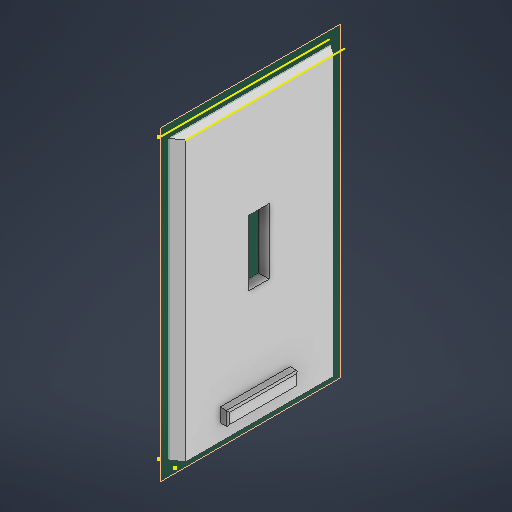
# Autodesk Inventor part: Part2
Saved by Autodesk Inventor 2026.1 (Build 301233000, 233)
## iProperties
Created: 2025-08-25
Part Number: Part2
Material: Generic
Document SubType Name: Modeling
Designer: usman
Density: 1 g/cm^3
Appearance: Default
Author: usman
Autodesk Inventor part; units mm, degrees
ref_plane "YZ Plane" through (0, 0, 0) normal (1, 0, 0) x (0, 1, 0)
ref_plane "XZ Plane" through (0, 0, 0) normal (0, 1, 0) x (-1, 0, 0)
ref_plane "XY Plane" through (0, 0, 0) normal (0, 0, 1) x (1, 0, 0)
sketch "Sketch1" plane through (0, 0, 0) normal (1, 0, 0) x (0, 1, 0)
  line L0 (0, 0) -> (178.9, 0)
  line L1 (178.9, 0) -> (178.9, -109)
  line L2 (178.9, -109) -> (0, -109)
  line L3 (0, -109) -> (0, 0)
  dimension "d0" = 178.9
  dimension "d1" = 109
  constraints: 8 end point, 2 parallel, 1 horizontal, 1 perpendicular
  measures "d0" distance of L1.end L2.end
  measures "d1" distance of L0.end L1.end
extrude "Extrusion1" add sketch "Sketch1" along normal blind 10
sketch "Sketch2" plane through (0, 178.9, 0) normal (0, 1, 0) x (1, 0, 0)
  point P0 (0, 0)
sketch "Sketch3" plane through (0, 178.9, 0) normal (0, 1, 0) x (1, 0, 0)
  line L0 (0, 109) -> (10, 101.9979)
  line L1 (10, 109) -> (10, 0) projected
  line L2 (0, 109) -> (0, 0) projected
  line L3 (0, 0) -> (10, 0) projected
  line L4 (0, 0) -> (10, 7.0021)
  dimension "d4" = 125
  dimension "d5" = 125
  constraints: 4 end point, 2 point on line
  measures "d4" angle of L2 L0
  measures "d5" angle of L2 L4
extrude "Extrusion2" cut sketch "Sketch3" against normal through all contours L4 L1 L3
sketch "Sketch4" plane through (0, 178.9, -109) normal (0, 1, 0) x (1, 0, 0)
  point P0 (0, -109)
sketch "Sketch5" plane through (0, 178.9, -109) normal (0, 1, 0) x (1, 0, 0)
  line L0 (0, -109) -> (0, 0) projected
  line L1 (10, 0) -> (10, -101.9979) projected
sketch "Sketch6" plane through (0, 178.9, -109) normal (0, 1, 0) x (1, 0, 0)
  line L0 (0, -109) -> (0, 0) projected
  line L1 (0, 0) -> (10, -7.0021)
  line L2 (10, 0) -> (10, -101.9979) projected
  line L3 (0, 0) -> (10, 0)
  line L4 (0, 0) -> (10, 0) projected
  line L5 (10, 0) -> (10, -7.0021)
  dimension "d8" = 125
  constraints: 6 end point, 1 collinear, 1 perpendicular, 1 point on line
  measures "d8" angle of L2 L1
extrude "Extrusion3" cut sketch "Sketch6" against normal through all
sketch "Sketch7" plane through (10, 0, 0) normal (1, 0, 0) x (0, 0, -1)
  point P0 (0, 0)
sketch "Sketch8" plane through (10, 0, 0) normal (1, 0, 0) x (0, 0, -1)
  line L0 (47.4589, 116.9) -> (60.4589, 116.9)
  line L1 (60.4589, 116.9) -> (60.4589, 74.9)
  line L2 (60.4589, 74.9) -> (47.4589, 74.9)
  line L3 (47.4589, 74.9) -> (47.4589, 116.9)
  line L4 (101.9979, 178.9) -> (7.0021, 178.9) projected
  point P0 (0, 0)
  dimension "d11" = 13
  dimension "d12" = 42
  dimension "d13" = 62
  constraints: 8 end point, 2 parallel, 1 horizontal, 1 perpendicular
  measures "d11" distance of L0.start L0.end
  measures "d12" distance of L0.end L1.end
  measures "d13" distance between parallel lines of L0 L4
extrude "Extrusion4" cut sketch "Sketch8" against normal through all
sketch "Sketch9" plane through (0, 0, 0) normal (0.5735764, 0, 0.819152) x (0.819152, 0, -0.5735764)
  point P0 (0, 0)
sketch "Sketch10" plane through (0, 0, 0) normal (0.5735764, 0, 0.819152) x (0.819152, 0, -0.5735764)
  point P0 (0, 0)
sketch "Sketch11" plane through (0, 178.9, 0) normal (0, 1, 0) x (1, 0, 0)
  line L0 (0, 109) -> (0, 0) projected
  line L1 (0, 109) -> (0.5, 109)
  line L2 (0.5, 109) -> (0.5, 0)
  line L3 (0.5, 0) -> (0, 0)
  line L4 (0, 0) -> (0, 109)
  dimension "d16" = 0.5
  constraints: 8 end point, 2 parallel, 1 horizontal, 1 perpendicular
  measures "d16" distance of L2.end L3.end
extrude "Extrusion5" cut sketch "Sketch11" against normal through all
sketch "Sketch12" plane through (10, 0, 0) normal (1, 0, 0) x (0, 0, -1)
  line L0 (73.9981, 10.7247) -> (29.0021, 10.7247)
  line L1 (29.0021, 10.7247) -> (29.0021, 19.4458)
  line L2 (29.0021, 19.4458) -> (73.9981, 19.4458)
  line L3 (73.9981, 19.4458) -> (73.9981, 10.7247)
  line L4 (7.0021, 178.9) -> (7.0021, 0) projected
  point P0 (0, 0)
  point P1 (29.0021, 15.0853)
  dimension "d19" = 22
  dimension "d20" = 44.996
  constraints: 8 end point, 2 parallel, 1 horizontal, 1 midpoint, 1 perpendicular
  measures "d19" distance from line of L4 point (29.002, 15.085)
  measures "d20" distance of L0.start L0.end
extrude "Extrusion6" add sketch "Sketch12" along normal blind 5
fillet "Fillet1" radius 1 4 edges at (15, 19.4458, -51.5001) (15, 10.7247, -51.5001) (15, 15.0853, -29.0021) (15, 15.0853, -73.9981)
sketch "Sketch14" plane through (10, 178.9, -7.0021) normal (0, 1, 0) x (1, 0, 0)
  line L0 (0, 94.9958) -> (-9.5, 101.6478) projected
  line L1 (-9.5, 101.6478) -> (-7, 101.6478)
  line L2 (-7, 101.6478) -> (-7, -6.652)
  line L3 (-7, -6.652) -> (-9.5, -6.652)
  line L4 (-9.5, -6.652) -> (-9.5, 101.6478)
  point P0 (-10, -7.0021)
  dimension "d25" = 2.5
  constraints: 8 end point, 2 parallel, 1 horizontal, 1 perpendicular
  measures "d25" distance of L2.end L3.end
extrude "Extrusion7" cut sketch "Sketch14" against normal through all
ref_plane "Work Plane2" through (4, 178.9, -106.8994) normal (-1, 0, 0) x (0, 0, 1)
sketch "Sketch15" plane through (4, 178.9, -106.8994) normal (-1, 0, 0) x (0, 0, 1)
  arc A0 (103.1758, -166.633) -> (98.1758, -166.633) centre (100.6758, -166.633) ccw
  arc A1 (6.623, -166.633) -> (1.623, -166.633) centre (4.123, -166.633) ccw
  line L0 (104.7988, -178.9) -> (0, -178.9) projected
  line L1 (104.7988, 0) -> (104.7988, -178.9) projected
  line L2 (0, -178.9) -> (0, 0) projected
  line L3 (103.1758, -166.633) -> (98.1758, -166.633)
  line L4 (6.623, -166.633) -> (1.623, -166.633)
  point P0 (106.8994, -178.9)
  dimension "d29" = 12.267
  dimension "d30" = 12.267
  dimension "d31" = 4.123
  dimension "d32" = 4.123
  dimension "d33" = 5
  dimension "d34" = 5
  constraints: 4 end point, 4 point on circle, 2 centre point, 2 point on line, 1 horizontal
  measures "d29" distance from line of A0.centre L0
  measures "d30" distance from line of A1.centre L0
  measures "d31" distance from line of A0.centre L1
  measures "d32" distance from line of L2 A1.centre
  measures "d33" diameter of A0
  measures "d34" diameter of A1
revolve "Revolution1" add sketch "Sketch15" angle 360 about axis through (4, 12.267, -3.7236) along (0, 0, -1)
body "Solid1"
